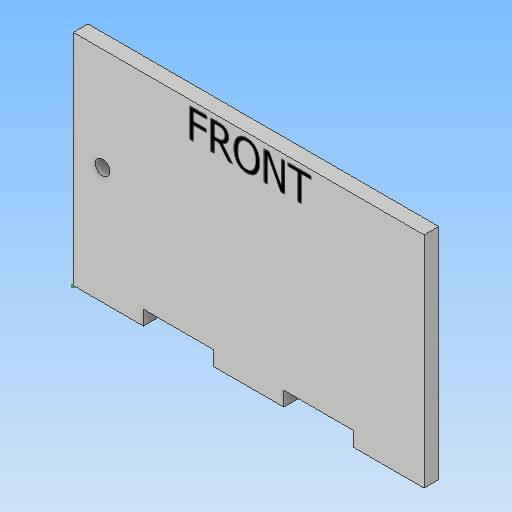
# Autodesk Inventor part: SpurGearMount
Saved by Autodesk Inventor 2017 (Build 210142000, 142)
## iProperties
Created: 2016-08-11
Part Number: SpurGearMount
Material: Generic
Document SubType Name: Modeling
Designer: Himesh Kurera
Density: 1 g/cm^3
Appearance: Default
Author: Himesh Kurera
Autodesk Inventor part; units mm, degrees
ref_plane "YZ Plane" through (0, 0, 0) normal (1, 0, 0) x (0, 1, 0)
ref_plane "XZ Plane" through (0, 0, 0) normal (0, 1, 0) x (-1, 0, 0)
ref_plane "XY Plane" through (0, 0, 0) normal (0, 0, 1) x (1, 0, 0)
sketch "Sketch1" plane through (0, 0, 0) normal (0, 0, 1) x (1, 0, 0)
  line L0 (0, 0) -> (120, 0)
  line L1 (120, 0) -> (120, 75)
  line L2 (120, 75) -> (0, 75)
  line L3 (0, 75) -> (0, 0)
  circle A0 centre (10, 40) radius 2.5
  dimension "d0" = 120
  dimension "d1" = 75
  dimension "d2" = 5
  dimension "d3" = 10
  dimension "d4" = 35
  constraints: 8 end point, 2 parallel, 1 centre point, 1 horizontal, 1 perpendicular
  measures "d0" distance of L2.end L1.end
  measures "d1" distance of L1.end L0.end
  measures "d2" diameter of A0
  measures "d3" distance from line of A0.centre L3
  measures "d4" distance from line of L2 A0.centre
extrude "Extrusion1" add sketch "Sketch1" along normal blind 5
sketch "Sketch2" plane through (0, 0, 5) normal (0, 0, 1) x (1, 0, 0)
  line L0 (0, 0) -> (120, 0) projected
  line L1 (24, 0) -> (48, 0)
  line L2 (48, 0) -> (48, 5)
  line L3 (48, 5) -> (24, 5)
  line L4 (24, 5) -> (24, 0)
  line L5 (72, 0) -> (96, 0)
  line L6 (96, 0) -> (96, 5)
  line L7 (96, 5) -> (72, 5)
  line L8 (72, 5) -> (72, 0)
  line L9 (0, 75) -> (0, 0) projected
  dimension "d7" = 24
  dimension "d8" = 5
  dimension "d9" = 24
  dimension "d10" = 5
  dimension "d11" = 24
  dimension "d12" = 24
  constraints: 16 end point, 4 parallel, 2 horizontal, 2 perpendicular, 2 point on line
  measures "d7" distance of L3.end L2.end
  measures "d8" distance of L2.end L1.end
  measures "d9" distance of L7.end L6.end
  measures "d10" distance of L6.end L5.end
  measures "d11" distance between parallel lines of L4 L9
  measures "d12" distance between parallel lines of L8 L2
extrude "Extrusion2" cut sketch "Sketch2" against normal blind 5
sketch "Sketch3" plane through (0, 0, 5) normal (0, 0, 1) x (1, 0, 0)
  line L0 (38.7826, 73.4019) -> (98.6345, 73.4019) construction
  line L1 (98.6345, 73.4019) -> (98.6345, 53.9975) construction
  line L2 (98.6345, 53.9975) -> (38.7826, 53.9975) construction
  line L3 (38.7826, 53.9975) -> (38.7826, 73.4019) construction
  point P0 (0, 0)
  constraints: 2 other
sketch "Sketch4" plane through (48, 0, 0) normal (0, -1, 0) x (1, 0, 0)
  line L0 (2.1203, 4.645) -> (24.7173, 4.645) construction
  line L1 (24.7173, 4.645) -> (24.7173, 0.4931) construction
  line L2 (24.7173, 0.4931) -> (2.1203, 0.4931) construction
  line L3 (2.1203, 0.4931) -> (2.1203, 4.645) construction
  point P0 (-48, 0)
  constraints: 2 other
sketch "Sketch5" plane through (0, 0, 0) normal (0, 0, -1) x (-1, 0, 0)
  line L0 (-77.429, 73.1669) -> (18.9429, 73.1669) construction
  line L1 (18.9429, 73.1669) -> (18.9429, 43.3318) construction
  line L2 (18.9429, 43.3318) -> (-77.429, 43.3318) construction
  line L3 (-77.429, 43.3318) -> (-77.429, 73.1669) construction
  point P0 (0, 0)
  constraints: 2 other
body "Solid1"
